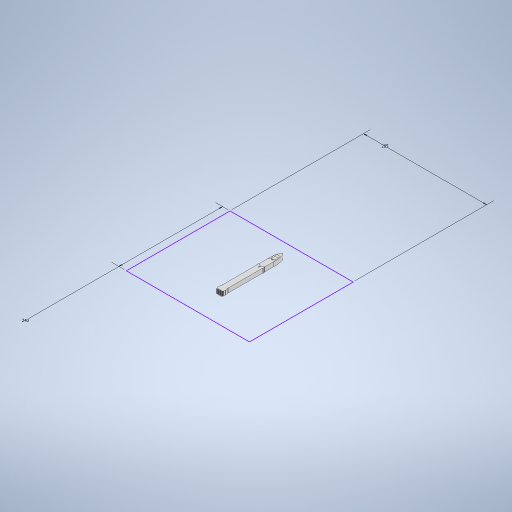
# Autodesk Inventor part: 2D-rocket-model
Saved by Autodesk Inventor 2024.1 (Build 281209000, 209)
## iProperties
Created: 2026-02-09
Part Number: 2D-rocket-model
Material: Generic
Document SubType Name: Modeling
Designer: iwheard
Density: 1 g/cm^3
Appearance: Default
Author: iwheard
Autodesk Inventor part; units mm, degrees
ref_plane "YZ Plane" through (0, 0, 0) normal (1, 0, 0) x (0, 1, 0)
ref_plane "XZ Plane" through (0, 0, 0) normal (0, 1, 0) x (-1, 0, 0)
ref_plane "XY Plane" through (0, 0, 0) normal (0, 0, 1) x (1, 0, 0)
sketch "Sketch3" plane through (0, 0, 0) normal (0, 1, 0) x (-1, 0, 0)
  line L0 (156.2321, -125.5014) -> (-128.7679, -125.5014)
  line L1 (-128.7679, -125.5014) -> (-128.7679, 114.4986)
  line L2 (-128.7679, 114.4986) -> (156.2321, 114.4986)
  line L3 (156.2321, 114.4986) -> (156.2321, -125.5014)
  point P0 (0, 0)
  dimension "d96" = 240
  dimension "d97" = 285
  constraints: 8 end point
  measures "d96" distance between parallel lines of L2 L0
  measures "d97" distance between parallel lines of L1 L3
sketch "Sketch1" plane through (0, 0, 0) normal (0, 1, 0) x (-1, 0, 0)
  line L0 (4.5, -41.85) -> (-4.5, -41.85)
  line L1 (-6.5, -41.85) -> (-6.5, 41.85)
  line L2 (-6.5, 41.85) -> (6.5, 41.85)
  line L3 (6.5, 41.85) -> (6.5, -41.85)
  line L4 (-6.5, -38.85) -> (-7.6, -38.85)
  line L5 (-7.6, -38.85) -> (-7.6, -41.85)
  line L6 (-7.6, -41.85) -> (-6.5, -41.85)
  line L7 (-6.5, -41.85) -> (-6.5, -38.85)
  line L8 (6.5, -38.85) -> (7.6, -38.85)
  line L9 (7.6, -38.85) -> (7.6, -41.85)
  line L10 (7.6, -41.85) -> (6.5, -41.85)
  line L11 (6.5, -41.85) -> (6.5, -38.85)
  line L12 (7.5, 41.85) -> (-7.5, 41.85)
  line L13 (-7.5, 41.85) -> (-7.5, 53.85)
  line L14 (-7.5, 53.85) -> (7.5, 53.85)
  line L15 (7.5, 53.85) -> (7.5, 41.85)
  line L16 (6.5, -41.85) -> (-6.5, -41.85)
  line L17 (-6.5, -43.85) -> (-6.5, -64.85)
  line L18 (-6.5, -64.85) -> (6.5, -64.85)
  line L19 (6.5, -64.85) -> (6.5, -43.85)
  line L20 (6.5, -64.85) -> (-6.5, -64.85)
  line L21 (-6.5, -64.85) -> (-6.5, -91.85) construction
  line L22 (-6.5, -91.85) -> (6.5, -91.85) construction
  line L23 (6.5, -91.85) -> (6.5, -64.85) construction
  line L24 (1.5, 53.85) -> (-1.5, 53.85)
  line L25 (-1.5, 53.85) -> (-1.5, 54.3639) construction
  line L26 (-1.5, 54.3639) -> (1.5, 54.3643) construction
  line L27 (1.5, 54.3643) -> (1.5, 53.85) construction
  line L28 (6.2, 53.85) -> (3.2, 53.85)
  line L29 (3.2, 53.85) -> (3.2, 54.3643) construction
  line L30 (3.2, 54.3643) -> (6.2, 54.3643) construction
  line L31 (6.2, 54.3643) -> (6.2, 53.85) construction
  line L32 (-3.2, 53.85) -> (-6.2, 53.85)
  line L33 (-6.2, 53.85) -> (-6.2, 54.3639)
  line L34 (-6.2, 54.3639) -> (-3.2, 54.3639) construction
  line L35 (-3.2, 54.3639) -> (-3.2, 53.85)
  line L36 (-6.2, 53.85) -> (-5.7688, 54.3639)
  line L37 (-5.7688, 54.3639) -> (-3.6312, 54.3639)
  line L38 (-3.6312, 54.3639) -> (-3.2, 53.85)
  line L39 (-1.5, 53.85) -> (-1.0688, 54.3639)
  line L40 (1.0685, 54.3643) -> (1.5, 53.85)
  line L41 (3.2, 53.85) -> (3.6312, 54.3643)
  line L42 (3.6312, 54.3643) -> (5.7688, 54.3643)
  line L43 (5.7688, 54.3643) -> (6.2, 53.85)
  line L44 (-1.0688, 54.3639) -> (1.0685, 54.3643)
  line L45 (-5.2885, 54.3639) -> (-5.5745, 54.7912) construction
  spline S0 degree 3 poles (-5.2885, 54.3639) (-5.5745, 54.7912) (-5.8233, 55.2234) (-5.9256, 55.9541) knots 1 1 1 1 2 2 2 2
  line L46 (-5.8233, 55.2234) -> (-5.9256, 55.9541) construction
  line L47 (-5.5745, 54.7912) -> (-5.8233, 55.2234) construction
  line L48 (-4.7, 54.3772) -> (-4.7, 58.1813)
  line L49 (0, 56.4172) -> (0, 60.7645)
  line L50 (4.7, 54.6227) -> (4.7, 58.7119)
  line L51 (-5.9256, 55.9541) -> (-5.8625, 56.0522) construction
  line L52 (-5.8625, 56.0522) -> (-4.7, 56.1293) construction
  spline S1 degree 2 poles (-5.9256, 55.9541) (-5.8625, 56.0522) (-4.7, 56.1293) knots 1 1 1 2 2 2
  line L53 (-4.1115, 54.3639) -> (-3.8255, 54.7912) construction
  spline S2 degree 3 poles (-4.1115, 54.3639) (-3.8255, 54.7912) (-3.5767, 55.2234) (-3.4744, 55.9541) knots 1 1 1 1 2 2 2 2
  line L54 (-3.5767, 55.2234) -> (-3.4744, 55.9541) construction
  line L55 (-3.8255, 54.7912) -> (-3.5767, 55.2234) construction
  line L56 (-3.4744, 55.9541) -> (-3.5375, 56.0522) construction
  line L57 (-3.5375, 56.0522) -> (-4.7, 56.1293) construction
  spline S3 degree 2 poles (-3.4744, 55.9541) (-3.5375, 56.0522) (-4.7, 56.1293) knots 1 1 1 2 2 2
  spline S4 degree 3 poles (-0.5885, 54.3639) (-0.8745, 54.7912) (-1.1233, 55.2234) (-1.2256, 55.9541) knots 1 1 1 1 2 2 2 2
  line L58 (-0.5885, 54.3639) -> (-0.8745, 54.7912) construction
  line L59 (-0.8745, 54.7912) -> (-1.1233, 55.2234) construction
  line L60 (-1.1233, 55.2234) -> (-1.2256, 55.9541) construction
  line L61 (-1.1625, 56.0522) -> (0, 56.1293) construction
  spline S5 degree 2 poles (-1.2256, 55.9541) (-1.1625, 56.0522) (0, 56.1293) knots 1 1 1 2 2 2
  line L62 (-1.2256, 55.9541) -> (-1.1625, 56.0522) construction
  line L63 (1.1625, 56.0522) -> (0, 56.1293) construction
  spline S6 degree 2 poles (1.2256, 55.9541) (1.1625, 56.0522) (0, 56.1293) knots 1 1 1 2 2 2
  line L64 (1.2256, 55.9541) -> (1.1625, 56.0522) construction
  spline S7 degree 3 poles (0.5885, 54.3639) (0.8745, 54.7912) (1.1233, 55.2234) (1.2256, 55.9541) knots 1 1 1 1 2 2 2 2
  line L65 (0.5885, 54.3639) -> (0.8745, 54.7912) construction
  line L66 (0.8745, 54.7912) -> (1.1233, 55.2234) construction
  line L67 (1.1233, 55.2234) -> (1.2256, 55.9541) construction
  spline S8 degree 3 poles (4.1115, 54.3639) (3.8255, 54.7912) (3.5767, 55.2234) (3.4744, 55.9541) knots 1 1 1 1 2 2 2 2
  line L68 (4.1115, 54.3639) -> (3.8255, 54.7912) construction
  line L69 (3.8255, 54.7912) -> (3.5767, 55.2234) construction
  line L70 (3.5767, 55.2234) -> (3.4744, 55.9541) construction
  line L71 (3.5375, 56.0522) -> (4.7, 56.1293) construction
  spline S9 degree 2 poles (3.4744, 55.9541) (3.5375, 56.0522) (4.7, 56.1293) knots 1 1 1 2 2 2
  line L72 (3.4744, 55.9541) -> (3.5375, 56.0522) construction
  line L73 (5.8625, 56.0522) -> (4.7, 56.1293) construction
  spline S10 degree 2 poles (5.9256, 55.9541) (5.8625, 56.0522) (4.7, 56.1293) knots 1 1 1 2 2 2
  line L74 (5.9256, 55.9541) -> (5.8625, 56.0522) construction
  spline S11 degree 3 poles (5.2885, 54.3639) (5.5745, 54.7912) (5.8233, 55.2234) (5.9256, 55.9541) knots 1 1 1 1 2 2 2 2
  line L75 (5.2885, 54.3639) -> (5.5745, 54.7912) construction
  line L76 (5.5745, 54.7912) -> (5.8233, 55.2234) construction
  line L77 (5.8233, 55.2234) -> (5.9256, 55.9541) construction
  line L78 (6.5, 41.85) -> (7.5, 47.85)
  line L79 (-6.5, 41.85) -> (-7.5, 47.85)
  line L80 (6.5, -64.85) -> (7, -74.5362) construction
  line L81 (7, -74.5362) -> (5.2352, -86.9996) construction
  line L82 (5.2352, -86.9996) -> (1.6435, -91.2819) construction
  line L83 (1.6435, -91.2819) -> (0, -91.6636) construction
  spline S12 degree 4 poles (6.5, -64.85) (7, -74.5362) (5.2352, -86.9996) (1.6435, -91.2819) (0, -91.6636) knots 1 1 1 1 1 2 2 2 2 2
  line L84 (-6.5, -64.85) -> (-7, -74.5362) construction
  line L85 (-7, -74.5362) -> (-5.2352, -86.9996) construction
  line L86 (-5.2352, -86.9996) -> (-1.6435, -91.2819) construction
  line L87 (-1.6435, -91.2819) -> (0, -91.6636) construction
  spline S13 degree 4 poles (-6.5, -64.85) (-7, -74.5362) (-5.2352, -86.9996) (-1.6435, -91.2819) (0, -91.6636) knots 1 1 1 1 1 2 2 2 2 2
  line L88 (1901.4999, -38.2925) -> (1902.9893, -38.2922)
  line L89 (1.1174, -35.6893) -> (0, -35.6371) construction
  spline S14 degree 2 poles (1.1744, -35.9047) (1.1174, -35.6893) (0, -35.6371) knots 1 1 1 2 2 2
  line L90 (1.1744, -35.9047) -> (1.1174, -35.6893) construction
  spline S15 degree 3 poles (0.3269, -38.204) (0.7855, -37.956) (1.2842, -36.908) (1.1744, -35.9047) knots 1 1 1 1 2 2 2 2
  line L91 (0.3269, -38.204) -> (0.7855, -37.956) construction
  line L92 (0.7855, -37.956) -> (1.2842, -36.908) construction
  line L93 (1.2842, -36.908) -> (1.1744, -35.9047) construction
  line L94 (0.3269, -38.204) -> (0.72, -38.2925)
  line L95 (0.72, -38.2925) -> (0.7855, -39.4293)
  line L96 (0.7855, -39.4293) -> (2.2488, -41.85)
  line L97 (0, -42.9416) -> (0, -40.7584)
  line L98 (-0.3269, -38.204) -> (-0.7855, -37.956) construction
  spline S16 degree 3 poles (-0.3269, -38.204) (-0.7855, -37.956) (-1.2842, -36.908) (-1.1744, -35.9047) knots 1 1 1 1 2 2 2 2
  line L99 (-0.7855, -37.956) -> (-1.2842, -36.908) construction
  line L100 (-1.2842, -36.908) -> (-1.1744, -35.9047) construction
  line L101 (-1.1174, -35.6893) -> (0, -35.6371) construction
  spline S17 degree 2 poles (-1.1744, -35.9047) (-1.1174, -35.6893) (0, -35.6371) knots 1 1 1 2 2 2
  line L102 (-1.1744, -35.9047) -> (-1.1174, -35.6893) construction
  line L103 (-0.3269, -38.204) -> (-0.72, -38.2925)
  line L104 (-0.72, -38.2925) -> (-0.7855, -39.4293)
  line L105 (-0.7855, -39.4293) -> (-2.2488, -41.85)
  line L106 (6.5, -64.85) -> (3.8744, -67.5271)
  line L107 (3.8744, -67.5271) -> (-3.8744, -67.5271)
  line L108 (-3.8744, -67.5271) -> (-6.5, -64.85)
  circle A0 centre (-2.2, -69.6931) radius 2.0154
  circle A1 centre (-3.7, -73.7175) radius 2.3319
  circle A2 centre (3.7, -73.7175) radius 2.3319
  circle A3 centre (2.2, -69.6931) radius 2.0154
  line L109 (1.75, -68.9208) -> (3.5, -75.8825)
  line L110 (3.5, -75.8825) -> (-3.5, -75.8825)
  line L111 (1.75, -68.9208) -> (-1.75, -68.9208)
  line L112 (-1.75, -68.9208) -> (-3.5, -75.8825)
  line L113 (0.35, -68.9208) -> (-0.35, -68.9208)
  line L114 (-0.35, -68.9208) -> (-0.35, -67.7212)
  line L115 (-0.3269, -67.6777) -> (0.3269, -67.6777)
  line L116 (0.35, -67.7212) -> (0.35, -68.9208)
  line L117 (0.3269, -67.6777) -> (0.2083, -67.5782) construction
  line L118 (0.2083, -67.5782) -> (0.1449, -67.4457) construction
  line L119 (0.1449, -67.4457) -> (0.6394, -67.0853) construction
  line L120 (0.6394, -67.0853) -> (1.0767, -66.0756) construction
  line L121 (1.0767, -66.0756) -> (1.1461, -65.608) construction
  spline S18 degree 4 poles (0.3269, -67.6777) (0.2083, -67.5782) (0.1449, -67.4457) (0.6394, -67.0853) (1.0767, -66.0756) (1.1461, -65.608) knots 1 1 1 1 1 2 3 3 3 3 3
  line L122 (1.1461, -65.608) -> (0.982, -65.4564) construction
  line L123 (0.982, -65.4564) -> (0, -65.4422) construction
  spline S19 degree 2 poles (1.1461, -65.608) (0.982, -65.4564) (0, -65.4422) knots 1 1 1 2 2 2
  line L124 (0.3269, -67.6777) -> (0.35, -67.6999) construction
  line L125 (0.35, -67.6999) -> (0.35, -67.7212) construction
  spline S20 degree 2 poles (0.3269, -67.6777) (0.35, -67.6999) (0.35, -67.7212) knots 1 1 1 2 2 2
  line L126 (-0.3269, -67.6777) -> (-0.2083, -67.5782) construction
  line L127 (-0.2083, -67.5782) -> (-0.1449, -67.4457) construction
  line L128 (-0.1449, -67.4457) -> (-0.6394, -67.0853) construction
  line L129 (-0.6394, -67.0853) -> (-1.0767, -66.0756) construction
  line L130 (-1.0767, -66.0756) -> (-1.1461, -65.608) construction
  spline S21 degree 4 poles (-0.3269, -67.6777) (-0.2083, -67.5782) (-0.1449, -67.4457) (-0.6394, -67.0853) (-1.0767, -66.0756) (-1.1461, -65.608) knots 1 1 1 1 1 2 3 3 3 3 3
  line L131 (-1.1461, -65.608) -> (-0.982, -65.4564) construction
  line L132 (-0.982, -65.4564) -> (0, -65.4422) construction
  spline S22 degree 2 poles (-1.1461, -65.608) (-0.982, -65.4564) (0, -65.4422) knots 1 1 1 2 2 2
  line L133 (3.5, -75.8825) -> (2.4833, -76.5825)
  line L134 (2.4833, -76.5825) -> (-2.4833, -76.5825)
  line L135 (-2.4833, -76.5825) -> (-3.5, -75.8825)
  line L136 (-0.3269, -67.6777) -> (-0.35, -67.6999) construction
  line L137 (-0.35, -67.6999) -> (-0.35, -67.7212) construction
  spline S23 degree 2 poles (-0.3269, -67.6777) (-0.35, -67.6999) (-0.35, -67.7212) knots 1 1 1 2 2 2
  line L138 (-0.1207, -68.0868) -> (-0.2854, -67.9502)
  line L139 (-0.2854, -67.9502) -> (-1.1545, -68.9978)
  line L140 (-1.1545, -68.9978) -> (-0.9898, -69.1344)
  line L141 (-0.9898, -69.1344) -> (-0.1207, -68.0868)
  line L142 (0.1207, -68.0868) -> (0.2854, -67.9502)
  line L143 (0.2854, -67.9502) -> (1.1545, -68.9978)
  line L144 (1.1545, -68.9978) -> (0.9898, -69.1344)
  line L145 (0.9898, -69.1344) -> (0.1207, -68.0868)
  line L146 (3.6383, -82.3131) -> (-3.6012, -82.3131)
  line L147 (-3.9012, -82.0131) -> (-3.9012, -76.8825)
  line L148 (-3.6012, -76.5825) -> (3.6383, -76.5825)
  line L149 (3.9383, -76.8825) -> (3.9383, -82.0131)
  line L150 (3.9383, -82.0131) -> (3.6383, -82.3131)
  line L151 (-3.6012, -82.3131) -> (-3.9012, -82.0131)
  line L152 (-3.6012, -76.5825) -> (-3.9012, -76.8825)
  line L153 (3.6383, -76.5825) -> (3.9383, -76.8825)
  line L154 (6.5, -43.85) -> (4.5, -41.85)
  line L155 (-4.5, -41.85) -> (-6.5, -43.85)
  line L156 (-6.5, -43.85) -> (-6.5, -41.85)
  line L157 (6.5, -43.85) -> (6.5, -41.85)
  spline S24 degree 5 poles (6.2004, -64.8655) (6.2594, -66.0095) (6.287, -67.1551) (6.2878, -68.3009) (6.2393, -70.5969) (6.0933, -72.8888) (5.9962, -74.0356) (5.7637, -76.2289) (5.4362, -78.4099) (5.2567, -79.4494) (4.8803, -81.355) (4.4067, -83.2385) (4.1677, -84.0932) (3.7006, -85.5877) (3.1329, -87.0465) (2.8649, -87.6693) (2.3739, -88.6911) (1.7817, -89.6566) (1.5238, -90.0312) (1.102, -90.5697) (0.5932, -91.0252) (0.4126, -91.16) (0.2161, -91.2848) (0, -91.3527) knots 0 0 0 0 0 0 0.204709 0.204709 0.204709 0.410312 0.410312 0.410312 0.598763 0.598763 0.598763 0.757291 0.757291 0.757291 0.878375 0.878375 0.878375 0.959518 0.959518 0.959518 1 1 1 1 1 1
  spline S25 degree 5 poles (0, -91.3527) (-0.2161, -91.2848) (-0.4126, -91.16) (-0.5932, -91.0252) (-1.102, -90.5697) (-1.5238, -90.0312) (-1.7817, -89.6566) (-2.3739, -88.6911) (-2.8649, -87.6693) (-3.1329, -87.0465) (-3.7006, -85.5877) (-4.1677, -84.0932) (-4.4067, -83.2385) (-4.8803, -81.355) (-5.2567, -79.4494) (-5.4362, -78.4099) (-5.7637, -76.2289) (-5.9962, -74.0356) (-6.0933, -72.8888) (-6.2393, -70.5969) (-6.2878, -68.3009) (-6.287, -67.1551) (-6.2594, -66.0095) (-6.2004, -64.8655) knots 0 0 0 0 0 0 0.040482 0.040482 0.040482 0.121625 0.121625 0.121625 0.242709 0.242709 0.242709 0.401237 0.401237 0.401237 0.589688 0.589688 0.589688 0.795291 0.795291 0.795291 1 1 1 1 1 1
  point P0 (0, 0)
  point P1 (7.05, -38.85)
  point P2 (0, 53.85)
  point P3 (0, 41.85)
  point P4 (0, 54.3641)
  point P5 (-6.2, 54.107)
  point P6 (0, 54.3641)
  point P7 (0, 53.85)
  point P8 (4.7, 54.3643)
  point P9 (4.7, 53.85)
  point P10 (-4.7, 54.3639)
  point P11 (4.7, 54.3643)
  point P12 (5.2888, 54.3643)
  point P13 (4.1112, 54.3643)
  point P14 (0.5887, 54.3642)
  point P15 (-0.5886, 54.364)
  point P16 (6.5, -38.85)
  point P17 (0, -41.85)
  point P18 (0, -41.85)
  point P19 (0, -41.85)
  point P20 (0, -64.85)
  point P21 (0, -64.85)
  point P22 (0, -67.6777)
  point P23 (0, -67.5271)
  point P24 (0, -67.6777)
  point P25 (0, -76.5825)
  point P26 (0, -75.8825)
  point P27 (-0.3269, -38.204)
  point P28 (-0.2307, -67.5271)
  point P29 (0.2307, -67.5271)
  point P30 (2.5792, -71.6725)
  point P31 (2.4594, -71.7429)
  point P32 (2.447, -71.6934)
  point P33 (0.3384, -68.9208)
  point P34 (0.35, -68.8935)
  point P35 (0.35, -68.3632)
  point P36 (0.5243, -68.5733)
  point P37 (-0.5243, -68.5733)
  point P38 (-0.35, -68.3632)
  point P39 (-0.35, -68.8935)
  point P40 (-0.3384, -68.9208)
  point P41 (3.2089, -71.4379)
  point P42 (0.6564, -68.3973)
  point P43 (0.35, -68.028)
  point P44 (-0.35, -68.028)
  point P45 (-0.6564, -68.3973)
  point P46 (-3.2089, -71.4379)
  point P47 (-3.3062, -76.0159)
  point P48 (3.3062, -76.0159)
  point P49 (-2.4594, -71.7429)
  point P50 (-2.5792, -71.6725)
  point P51 (-2.447, -71.6934)
  point P52 (3.9383, -82.3131)
  point P53 (-3.9012, -76.5825)
  point P54 (-3.9012, -82.3131)
  point P55 (3.9383, -76.5825)
  point P56 (6.2139, -65.1417)
  point P57 (6.0255, -73.5448)
  point P58 (-6.0255, -73.5448)
  point P59 (-6.2139, -65.1417)
  point P60 (6.5, -41.85)
  point P61 (-6.5, -41.85)
  point P62 (0, -38.3845)
  point P63 (0, -38.7745)
  dimension "d82" = 0.3
  dimension "d0" = 83.7
  dimension "d1" = 13
  dimension "d2" = 6.5
  dimension "d3" = 41.85
  dimension "d4" = 3
  dimension "d5" = 1.1
  dimension "d6" = 1.1
  dimension "d7" = 12
  dimension "d8" = 15
  dimension "d9" = 23
  dimension "d10" = 1
  dimension "d11" = 1
  dimension "d12" = 27
  dimension "d13" = 3
  dimension "d14" = 3
  dimension "d15" = 3
  dimension "d16" = 1.3
  dimension "d17" = 1.3
  dimension "d18" = 1.7
  dimension "d19" = 1.7
  dimension "d20" = 50
  dimension "d21" = 50
  dimension "d22" = 2.1375
  dimension "d24" = 2.1375
  dimension "d26" = 50
  dimension "d28" = 50
  dimension "d31" = 4.7
  dimension "d36" = 6
  dimension "d57" = 2.2
  dimension "d58" = 2.2
  dimension "d59" = 3.7
  dimension "d60" = 3.7
  dimension "d61" = 0.35
  dimension "d62" = 0.35
  dimension "d63" = 1.4
  dimension "d64" = 1.4
  dimension "d65" = 3.5
  dimension "d66" = 3.5
  dimension "d67" = 0.7
  dimension "d72" = 0.3
  dimension "d73" = 0.3
  dimension "d74" = 0.3
  dimension "d75" = 0.3
  dimension "d76" = 0.3
  dimension "d77" = 0.3
  dimension "d78" = 0.3
  dimension "d79" = 0.3
  dimension "d90" = 2
  dimension "d91" = 2
  dimension "d92" = 2
  dimension "d93" = 2
  constraints: 184 end point, 33 symmetric about line, 31 horizontal alignment, 22 midpoint, 18 point on line, 18 vertical alignment, 11 horizontal, 6 coincident, 4 centre point, 4 vertical, 2 equal radius, 120 other
  measures "d0" distance between parallel lines of L2 L0
  measures "d1" distance between parallel lines of L1 L3
  measures "d2" distance from line of point (0, 0) L3
  measures "d3" distance from line of L2 point (0, 0)
  measures "d4" distance between parallel lines of L4 L6
  measures "d5" distance between parallel lines of L5 L1
  measures "d6" distance between parallel lines of L9 L3
  measures "d7" distance between parallel lines of L14 L12
  measures "d8" distance between parallel lines of L13 L15
  measures "d9" distance between parallel lines of L0 L18
  measures "d10" distance between parallel lines of L3 L15
  measures "d11" distance between parallel lines of L1 L13
  measures "d12" distance between parallel lines of L18 L22
  measures "d13" distance between parallel lines of L29 L31
  measures "d14" distance between parallel lines of L25 L27
  measures "d15" distance between parallel lines of L33 L35
  measures "d16" distance between parallel lines of L15 L31
  measures "d17" distance from line of point (-6.2, 54.107) L13
  measures "d18" distance between parallel lines of L27 L29
  measures "d19" distance between parallel lines of L35 L25
  measures "d20" angle of L14 L36
  measures "d21" angle of L32 L38
  measures "d22" distance of L37.end L36.end
  measures "d24" distance of L42.end L41.end
  measures "d26" angle of L24 L39
  measures "d28" angle of L24 L40
  measures "d31" distance of L45.start L58.start
  measures "d36" distance of L14.end L78.end
  measures "d57" horizontal distance of point (0, -64.85) A3.centre
  measures "d58" horizontal distance of point (0, -64.85) A0.centre
  measures "d59" horizontal distance of point (0, -64.85) A2.centre
  measures "d60" horizontal distance of point (0, -64.85) A1.centre
  measures "d61" distance from line of L116 point (0, -67.527)
  measures "d62" distance from line of point (0, -67.678) L114
  measures "d63" distance from line of L109.start L116
  measures "d64" distance from line of L111.end L114
  measures "d65" horizontal distance of point (0, -67.678) L109.end
  measures "d66" horizontal distance of point (0, -67.678) L110.end
  measures "d67" distance between parallel lines of L134 L110
  measures "d72" distance of L149.end point (3.938, -82.313)
  measures "d73" distance of L146.start point (3.938, -82.313)
  measures "d74" distance of L146.end point (-3.901, -82.313)
  measures "d75" distance of L147.start point (-3.901, -82.313)
  measures "d76" distance of L148.start point (-3.901, -76.582)
  measures "d77" distance of L147.end point (-3.901, -76.582)
  measures "d78" distance of L148.end point (3.938, -76.582)
  measures "d79" distance of L149.start point (3.938, -76.582)
  measures "d90" distance of L19.end point (6.5, -41.85)
  measures "d91" distance of L0.start point (6.5, -41.85)
  measures "d92" distance of L0.end point (-6.5, -41.85)
  measures "d93" distance of L17.start point (-6.5, -41.85)
extrude "Extrusion1" add sketch "Sketch1" along normal blind 10 contours L0 L96 L95 L94 S15 S14 S17 S16 L103 L104 L105 L16 L1 L2 L3 | L16 L157 L154 | L3 L8 L9 L10 | L2 L79 L13 L14 L15 L78 | L155 L156 L16 | L6 L5 L4 L1 | L14 L41 L42 L43 | L36 L37 L38 L14 | L14 L39 L44 L40 | L42 S8 S9 S10 S11 | S0 S1 S3 S2 L37 | L44 S4 S5 S6 S7
extrude "Extrusion2" add sketch "Sketch1" along normal blind 10 separate body contours L154 L19 L18 L17 L155 L0 | L0 L105 L104 L103 S16 S17 S14 S15 L94 L95 L96 | L106 L107 S18 S19 S22 S21 L108 L18 | L107 S21 S22 S19 S18
extrude "Extrusion3" add sketch "Sketch1" along normal blind 10 separate body contours S24 A2 L133 L109 A3 | A2 S24 | S25 A1 | A1 A0 L112 L135 S25 | S18 L115 S21 L107 | L107 S21 S22 S19 S18 | A3 A2 | A2 A3 L109 L111 L143 | A1 A0 | A0 L139 L111 L112 A1 | S20 L116 L143 L142 L145 A3 L111 A0 L114 L141 L138 L139 S23 L115 | L133 L134 L135 A1 L110 A2 | A2 L110 L133 | L139 L114 L141 A0 | A0 L141 L111 L139 | L135 L110 A1 | L109 L110 A2 | A2 L110 A1 L112 A0 L111 A3 L109 | A3 L111 L145 L144 L143 L109 | L143 L111 L145 A3 | A3 L145 L116 L143 | L141 L114 A0 | A0 L114 L111 L141 | L139 L138 L141 L114 | L139 L140 L141 L111 A0 L112 | L111 L141 L140 L139 | A1 L110 L112 | L116 L145 L142 L143 | A3 L116 L111 | L145 L111 L116 A3 | A3 L116 L145 | L143 L144 L145 L111 | A0 L111 L114
extrude "Extrusion4" add sketch "Sketch1" along normal blind 10 separate body contours L148 L153 L149 L150 L146 L151 L147 L152 L134
extrude "Extrusion5" add sketch "Sketch1" along normal blind 10 separate body contours S12 S13 L108 S25 A1 S24 A2 L106 | S24 A2 A3 L143 L116 S20 S18 L107 L106 | L108 L107 S21 S23 L114 L139 A0 A1 S25 | S24 S25 A1 L135 L148 L152 L147 L151 L146 L150 L149 L153 L133 A2
chamfer "Chamfer1" distance 0.5 distance2 1 1 edges at (7.6, 5, -41.85) measured on face at (7.6, 3.3333, -39.85)
chamfer "Chamfer2" distance 0.5 distance2 1 1 edges at (7.6, 5, -38.85) measured on face at (7.6, 3.3333, -39.6833)
chamfer "Chamfer3" distance 0.5 distance2 1 1 edges at (-7.6, 5, -41.85) measured on face at (-7.6, 3.3333, -40.85)
chamfer "Chamfer4" distance 0.5 distance2 1 1 edges at (-7.6, 5, -38.85) measured on face at (-7.6, 3.3333, -40.5167)
chamfer "Chamfer5" distance 1 angle 45 2 edges at (7.5, 5, 53.85) (-7.5, 5, 53.85)
fillet "Fillet1" radius 1 4 edges at (-7.5, 5, 52.85) (-6.5, 5, 53.85) (6.5, 5, 53.85) (7.5, 5, 52.85)
fillet "Fillet2" radius 4 4 edges at (7.5, 5, 47.85) (6.5, 5, 41.85) (-7.5, 5, 47.85) (-6.5, 5, 41.85)
equation "\"d2\" = 0.5 * d1"
equation "\"d3\" = 0.5 * d0"
equation "\"d6\" = d5"
equation "\"d24\" = d22"
body "Solid1"
body "Solid2"
body "Solid3"
body "Solid4"
body "Solid5"
